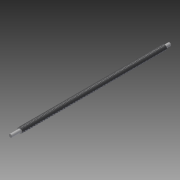
# Autodesk Inventor part: MTSBRW10-310-F18-V6-S10-Q6
Saved by Autodesk Inventor 2015 SP1 (Build 190203100, 203)
## iProperties
Category: Hardware
Created: 2014-01-02
Part Number: MTSBRW10-310-F18-V6-S10-Q6
Material: Steel
Document SubType Name: Modeling
Designer: Jack
Density: 7.85 g/cm^3
Appearance: Steel
Mass: 182.71 g
Surface Area: 96.2082 cm^2
Volume: 23.2751 cm^3
Vendor: Misumi
Catalog Web Link: http://us.misumi-ec.com/vona2/detail/110300083060
Stock Number: MTSBRW10-310-F18-V6-S10-Q6
Author: Jack
Title: Z Axis Lead Screw
Autodesk Inventor part; units mm, degrees
ref_plane "YZ Plane" through (0, 0, 0) normal (1, 0, 0) x (0, 1, 0)
ref_plane "XZ Plane" through (0, 0, 0) normal (0, 1, 0) x (-1, 0, 0)
ref_plane "XY Plane" through (0, 0, 0) normal (0, 0, 1) x (1, 0, 0)
sketch "Sketch1" plane through (0, 0, 0) normal (0, 1, 0) x (-1, 0, 0)
  circle A0 centre (0, 0) radius 3
  dimension "d0" = 6
  constraints: 1 centre point, 1 coincident
  measures "d0" diameter of A0
extrude "Extrusion1" add sketch "Sketch1" along normal blind 18
sketch "Sketch5" plane through (0, 18, 0) normal (0, 1, 0) x (1, 0, 0)
  circle A0 centre (0, 0) radius 3 projected
  circle A1 centre (0, 0) radius 5
  dimension "d20" = 10
  constraints: 1 centre point, 1 coincident
  measures "d20" diameter of A1
extrude "Extrusion5" add sketch "Sketch5" along normal blind 282 contours A0 | A1
sketch "Sketch6" plane through (0, 300, 0) normal (0, 1, 0) x (1, 0, 0)
  circle A0 centre (0, 0) radius 5 projected
  circle A1 centre (0, 0) radius 3
  dimension "d23" = 6
  constraints: 1 centre point, 1 coincident
  measures "d23" diameter of A1
extrude "Extrusion6" add sketch "Sketch6" along normal blind 10 contours A1
thread "Thread2" size "M10x1.5" class "6g" standard "ANSI Metric M Profile" full length
thread "Thread3" size "TR10x1.5" class "7e" standard "ISO Metric Trapezoidal Threads" full length
body "Solid1"
